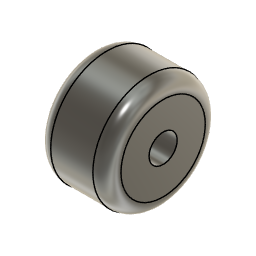
FlyWheel-Bot v1 (Autodesk Fusion 360 design; units mm, degrees)
Autodesk Fusion 360 part; units mm, degrees
sketch "Sketch1" plane through (0, 0, 0) normal (1, 0, 0) x (0, 1, 0)
  circle A0 centre (0, 0) radius 1
  circle A1 centre (0, 0) radius 4
  dimension "d1" = 2
  dimension "d2" = 8
  constraint coincident A0.centre A1.centre
  measures "d1" diameter of A0
  measures "d2" diameter of A1
extrude "Extrude1" add sketch "Sketch1" along normal blind 5
fillet "Fillet1" radius 1 1 edges at (0, -3.7293, -1.4465)
fillet "Fillet2" radius 1 1 edges at (5, -3.7293, -1.4465)
